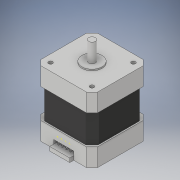
# Autodesk Inventor part: Nema17drylin
Saved by Autodesk Inventor 2021.3 (Build 253353000, 353)
## iProperties
Created: 2020-01-07
Part Number: Nema17drylin
Material: Generisch
Document SubType Name: Modeling
Designer: kaebi
Density: 1 g/cm^3
Appearance: Vorgabe
Description: y-Motor (Bestand)
Stock Number: -
Author: kaebi
Autodesk Inventor part; units mm, degrees
ref_plane "YZ Plane" through (0, 0, 0) normal (1, 0, 0) x (0, 1, 0)
ref_plane "XZ Plane" through (0, 0, 0) normal (0, 1, 0) x (-1, 0, 0)
ref_plane "XY Plane" through (0, 0, 0) normal (0, 0, 1) x (1, 0, 0)
sketch "Skizze1" plane through (0, 0, 0) normal (0, 1, 0) x (-1, 0, 0)
  line L0 (-21.15, 21.15) -> (21.15, 21.15)
  line L1 (21.15, 21.15) -> (21.15, -21.15)
  line L2 (21.15, -21.15) -> (-21.15, -21.15)
  line L3 (-21.15, -21.15) -> (-21.15, 21.15)
  line L4 (-21.15, 21.15) -> (21.15, -21.15) construction
  line L5 (21.15, 21.15) -> (-21.15, -21.15) construction
  point P0 (0, 0)
  dimension "d0" = 42.3
  dimension "d1" = 42.3
  constraints: 12 end point, 2 midpoint, 2 parallel, 1 horizontal, 1 perpendicular
  measures "d0" distance of L0.end L1.end
  measures "d1" distance of L1.end L2.end
extrude "Extrusion1" add sketch "Skizze1" along normal mid plane 49
sketch "Skizze2" plane through (0, -24.5, 0) normal (0, -1, 0) x (1, 0, 0)
  line L0 (-21.15, 21.15) -> (21.15, 21.15) projected
  line L1 (-7.5, 21.15) -> (7.5, 21.15)
  line L2 (7.5, 21.15) -> (7.5, 24.15)
  line L3 (7.5, 24.15) -> (-7.5, 24.15)
  line L4 (-7.5, 24.15) -> (-7.5, 21.15)
  line L5 (0, -30.21) -> (0, 33.21) projected
  point P0 (0, 0)
  dimension "d4" = 15
  dimension "d5" = 3
  constraints: 8 end point, 2 parallel, 1 horizontal, 1 perpendicular, 1 point on line, 1 other
  measures "d4" distance of L2.end L3.end
  measures "d5" distance of L1.end L2.end
extrude "Extrusion2" add sketch "Skizze2" against normal blind 3
sketch "Skizze3" plane through (0, -24.5, 0) normal (0, -1, 0) x (1, 0, 0)
  line L0 (-15.5, -15.5) -> (15.5, -15.5)
  line L1 (15.5, -15.5) -> (15.5, 15.5)
  line L2 (15.5, 15.5) -> (-15.5, 15.5)
  line L3 (-15.5, 15.5) -> (-15.5, -15.5)
  line L4 (-15.5, -15.5) -> (15.5, 15.5) construction
  line L5 (15.5, -15.5) -> (-15.5, 15.5) construction
  circle A0 centre (-15.5, 15.5) radius 1.5
  circle A1 centre (15.5, 15.5) radius 1.5
  circle A2 centre (15.5, -15.5) radius 1.5
  circle A3 centre (-15.5, -15.5) radius 1.5
  circle A4 centre (0, 0) radius 4.5
  dimension "d8" = 31
  dimension "d9" = 31
  dimension "d10" = 3
  dimension "d11" = 9
  constraints: 12 end point, 5 centre point, 5 coincident, 3 equal radius, 2 midpoint, 2 parallel, 1 horizontal, 1 perpendicular
  measures "d8" distance of L2.end L1.end
  measures "d9" distance of L1.end L0.end
  measures "d10" diameter of A0
  measures "d11" diameter of A4
extrude "Extrusion3" cut sketch "Skizze3" along normal through all both and the other way through all contours L3 A3 L0 | L0 A3 L3 | A2 L1 L0 | L0 L1 A2 | A0 L2 L3 | L3 L2 A0 | A1 L2 L1 | L1 L2 A1 | A4
chamfer "Fase1" distance 4 angle 45 4 edges at (21.15, 0, 21.15) (-21.15, 0, 21.15) (21.15, 0, -21.15) (-21.15, 0, -21.15)
sketch "Skizze4" plane through (0, 0, 0) normal (0, 1, 0) x (-1, 0, 0)
  line L0 (20.15, 15.3216) -> (15.3216, 20.15)
  line L1 (-15.3216, 20.15) -> (-20.15, 15.3216)
  line L2 (-20.15, -15.3216) -> (-15.3216, -20.15)
  line L3 (15.3216, -20.15) -> (20.15, -15.3216)
  line L4 (25.5, -25.5) -> (-25.5, -25.5)
  line L5 (-25.5, -25.5) -> (-25.5, 25.5)
  line L6 (-25.5, 25.5) -> (25.5, 25.5)
  line L7 (25.5, 25.5) -> (25.5, -25.5)
  line L8 (25.5, -25.5) -> (-25.5, 25.5) construction
  line L9 (-25.5, -25.5) -> (25.5, 25.5) construction
  line L10 (-21.15, 17.15) -> (-17.15, 21.15) projected
  line L11 (-17.15, -21.15) -> (-21.15, -17.15) projected
  line L12 (21.15, -17.15) -> (17.15, -21.15) projected
  line L13 (17.15, 21.15) -> (21.15, 17.15) projected
  line L14 (20.15, 15.3216) -> (20.15, -15.3216)
  line L15 (15.3216, -20.15) -> (-15.3216, -20.15)
  line L16 (-20.15, -15.3216) -> (-20.15, 15.3216)
  line L17 (-15.3216, 20.15) -> (15.3216, 20.15)
  line L18 (17.15, 21.15) -> (-17.15, 21.15) projected
  line L19 (-21.15, 17.15) -> (-21.15, -17.15) projected
  line L20 (-17.15, -21.15) -> (17.15, -21.15) projected
  line L21 (21.15, -17.15) -> (21.15, 17.15) projected
  point P0 (0, 0)
  dimension "d21" = 2
  dimension "d22" = 1
  dimension "d24" = 1
  dimension "d25" = 1
  constraints: 28 end point, 10 parallel, 10 perpendicular, 2 midpoint, 1 horizontal, 1 vertical
  measures "d21" distance between parallel lines of L10 L1
  measures "d22" distance between parallel lines of L18 L17
  measures "d24" distance between parallel lines of L21 L14
  measures "d25" distance between parallel lines of L20 L15
extrude "Extrusion4" cut sketch "Skizze4" along normal mid plane 22 contours L4 L5 L6 L7 | L10 L18 L13 L21 L12 L20 L11 L19
sketch "Skizze6" plane through (-7.5, -21.5, 21.15) normal (0, 0, 1) x (1, 0, 0)
  line L0 (0, 0) -> (15, 0)
  line L1 (15, 0) -> (15, 3)
  line L2 (15, 3) -> (0, 3)
  line L3 (0, 3) -> (0, 0)
  line L4 (15, -3) -> (15, 0) projected
  line L5 (0, -3) -> (0, 0) projected
  line L6 (0, 0) -> (15, 0) projected
  line L7 (2.5, 1) -> (3.5, 1)
  line L8 (3.5, 1) -> (3.5, 2)
  line L9 (3.5, 2) -> (2.5, 2)
  line L10 (2.5, 2) -> (2.5, 1)
  line L11 (2.5, 1) -> (3.5, 2) construction
  line L12 (3.5, 1) -> (2.5, 2) construction
  line L13 (5.5, 1) -> (6.5, 1)
  line L14 (6.5, 1) -> (6.5, 2)
  line L15 (6.5, 2) -> (5.5, 2)
  line L16 (5.5, 2) -> (5.5, 1)
  line L17 (5.5, 1) -> (6.5, 2) construction
  line L18 (6.5, 1) -> (5.5, 2) construction
  line L19 (8.5, 1) -> (9.5, 1)
  line L20 (9.5, 1) -> (9.5, 2)
  line L21 (9.5, 2) -> (8.5, 2)
  line L22 (8.5, 2) -> (8.5, 1)
  line L23 (8.5, 1) -> (9.5, 2) construction
  line L24 (9.5, 1) -> (8.5, 2) construction
  line L25 (11.5, 1) -> (12.5, 1)
  line L26 (12.5, 1) -> (12.5, 2)
  line L27 (12.5, 2) -> (11.5, 2)
  line L28 (11.5, 2) -> (11.5, 1)
  line L29 (11.5, 1) -> (12.5, 2) construction
  line L30 (12.5, 1) -> (11.5, 2) construction
  line L31 (7.5, -12.8) -> (7.5, 55.8) projected
  point P0 (7.5, 21.5)
  point P1 (3, 1.5)
  point P2 (6, 1.5)
  point P3 (9, 1.5)
  point P4 (12, 1.5)
  point P5 (12, 1.5)
  point P6 (15, 1.5)
  dimension "d29" = 3
  dimension "d30" = 3
  dimension "d31" = 3
  dimension "d32" = 1
  dimension "d33" = 1
  constraints: 56 end point, 10 midpoint, 10 parallel, 5 equal length, 5 horizontal, 5 perpendicular, 3 collinear, 2 point on line, 2 symmetric about line, 1 horizontal alignment
  measures "d29" distance of L0.end L1.end
  measures "d30" distance of point (6, 1.5) point (9, 1.5)
  measures "d31" distance of point (6, 1.5) point (3, 1.5)
  measures "d32" distance of L26.end L27.end
  measures "d33" distance of L25.end L26.end
extrude "Extrusion6" cut sketch "Skizze6" against normal blind 5
sketch "Skizze7" plane through (0, 0, 0) normal (1, 0, 0) x (0, 1, 0)
  line L0 (39.5, 0) -> (39.5, 2.5)
  line L1 (39.5, 2.5) -> (25.5, 2.5)
  line L2 (25.5, 2.5) -> (25.5, 7.5)
  line L3 (25.5, 7.5) -> (24.5, 7.5)
  line L4 (24.5, -17.15) -> (24.5, 17.15) projected
  line L5 (24.5, 0) -> (39.5, 0)
  line L6 (24.5, 0) -> (24.5, 7.5)
  line L7 (38.5419, 0) -> (33.7383, 0)
  point P0 (0, 0)
  dimension "d37" = 5
  dimension "d38" = 1
  dimension "d39" = 15
  dimension "d40" = 15
  constraints: 14 end point, 3 perpendicular, 2 collinear, 1 horizontal, 1 midpoint, 1 parallel, 1 point on line, 1 vertical
  measures "d37" diameter of L1 L7
  measures "d38" distance of L2.end L3.end
  measures "d39" diameter of L3 L7
  measures "d40" distance between parallel lines of L4 L0
revolve "Umdrehung1" add sketch "Skizze7" angle 360 about axis through (0, 24.5, 0) along (0, 1, 0)
equation "\"d24\" = d22"
equation "\"d25\" = d22"
equation "\"d31\" = d30"
equation "\"d33\" = d32"
